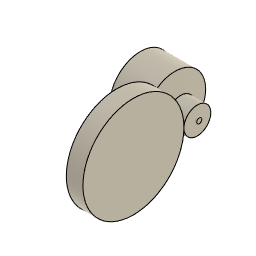
Gondel (Autodesk Fusion 360 design; units mm, degrees)
Autodesk Fusion 360 part; units mm, degrees
sketch "Skizze1" plane through (0, 0, 0) normal (0, 0, 1) x (1, 0, 0)
  circle A0 centre (0, 0) radius 12
  dimension "d1" = 24
  constraint coincident A0.centre origin
  measures "d1" diameter of A0
extrude "Extrusion1" add sketch "Skizze1" along normal blind 13.5 makes body 1
sketch "Skizze2" plane through (0, 0, 13.5) normal (0, 0, 1) x (-1, 0, 0)
sketch "Skizze3" plane through (0, 0, 13.5) normal (0, 0, 1) x (-1, 0, 0)
  circle A0 centre (0, 0) radius 1
  dimension "d5" = 2
  constraint coincident A0.centre origin
  measures "d5" diameter of A0
extrude "Extrusion2" add sketch "Skizze3" along normal blind 14.5 bodies 1
extrude "Extrusion3" cut 1 faces at (0.3296, -0.5031, 28) along direction (0, 0, -1) blind 10 on bodies 1 bodies 1
extrude "Extrusion4" add 1 faces at (0.3296, -0.5031, 18) along direction (0, 0, 1) blind 5 on bodies 1 bodies 1
sketch "Skizze4" plane through (0, 0, 0) normal (0, 1, 0) x (1, 0, 0)
sketch "Skizze5" plane through (0, 0, 13.5) normal (0, 0, 1) x (-1, 0, 0)
sketch "Skizze6" plane through (0, 0, 0) normal (0, 0, 1) x (1, 0, 0)
  circle A0 centre (0, 0) radius 5.25
  dimension "d12" = 10.5
  constraint coincident A0.centre origin
  measures "d12" diameter of A0
extrude "Extrusion5" add sketch "Skizze6" along normal blind 6.5 separate body makes body 2
sketch "Skizze7" plane through (0, 0, 0) normal (0, 1, 0) x (1, 0, 0)
  circle A0 centre (0, 0) radius 19.75
  dimension "d15" = 39.5
  constraint coincident A0.centre origin
  measures "d15" diameter of A0
extrude "Extrusion6" add sketch "Skizze7" along normal blind 6.5 separate body makes body 3
move_body "Verschieben1" bodies 3 to x (1, 0, 0) y (0, 1, 0) z (0, 0, 1) at (30, 0, 0)
move_body "Verschieben2" bodies 1 to x (1, 0, 0) y (0, 1, 0) z (0, 0, 1) at (-25, 0, 0)
move_body "Verschieben3" bodies 1 to x (0, 0, -1) y (0, 1, 0) z (1, 0, 0) at (-37, 0, -37)
move_body "Verschieben4" bodies 2 to x (0, 0, -1) y (0, 1, 0) z (1, 0, 0) at (-21.25, 0, -12.25)
copy_body "Körper->Berechn1" bodies 1 removing the originals makes body 4 in component "Motor"
copy_body "Körper->Berechn2" bodies 2 removing the originals makes body 5 in component "Kleines Zahnrad"
move_body "Verschieben5" bodies 3 to x (0, 1, 0) y (-1, 0, 0) z (0, 0, 1) at (10.25, -10.25, 0)
move_body "Verschieben6" bodies 3 to x (1, 0, 0) y (0, 1, 0) z (0, 0, 1) at (0, -19, 0)
move_body "Verschieben7" bodies 3 to x (1, 0, 0) y (0, 1, 0) z (0, 0, 1) at (0, 20, 0)
move_body "Verschieben8" bodies 3 to x (1, 0, 0) y (0, 1, 0) z (0, 0, 1) at (0, -0.9, 0)
move_body "Verschieben9" bodies 3 to x (1, 0, 0) y (0, 1, 0) z (0, 0, 1) at (0, -0.1, 0)
move_body "Verschieben10" bodies 3 to x (1, 0, 0) y (0, 1, 0) z (0, 0, 1) at (0, -19.75, 0)
move_body "Verschieben1'" bodies 4 to x (1, 0, 0) y (0, 1, 0) z (0, 0, 1) at (0, 25, 0) in component "Motor"
move_body "Verschieben1''" bodies 5 to x (1, 0, 0) y (0, 1, 0) z (0, 0, 1) at (0, 25, 0) in component "Kleines Zahnrad"
move_body "Verschieben2'" bodies 4 to x (1, 0, 0) y (0, 1, 0) z (0, 0, 1) at (25, 0, 0) in component "Motor"
move_body "Verschieben2''" bodies 5 to x (1, 0, 0) y (0, 1, 0) z (0, 0, 1) at (25, 0, 0) in component "Kleines Zahnrad"
move_body "Verschieben3'" bodies 4 to x (1, 0, 0) y (0, 1, 0) z (0, 0, 1) at (0, 0, 12) in component "Motor"
move_body "Verschieben3''" bodies 5 to x (1, 0, 0) y (0, 1, 0) z (0, 0, 1) at (0, 0, 12) in component "Kleines Zahnrad"
component "Motor" placed x (1, 0, 0) y (0, 1, 0) z (0, 0, 1) at (0, 0, 0)
component "Kleines Zahnrad" placed x (1, 0, 0) y (0, 1, 0) z (0, 0, 1) at (0, 0, 0)
named bodies: "Motor", "Kleines Zahnrad", "Großes zahnrad"
